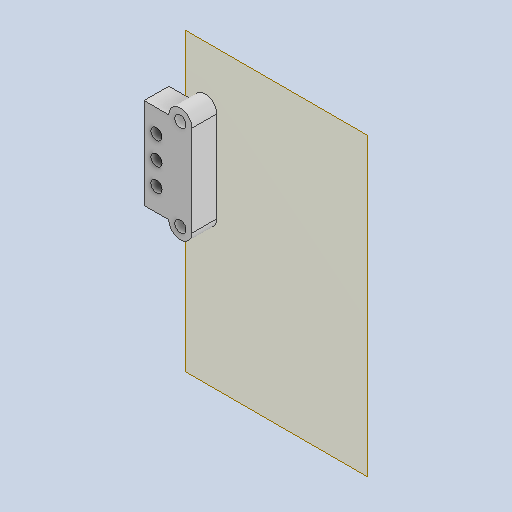
# Autodesk Inventor part: _idle_adt
Saved by Autodesk Inventor 2024.3 (Build 283343000, 343)
## iProperties
Created: 2024-09-05
Part Number: _idle_adt
Material: 일반
Document SubType Name: Modeling
Designer: gretc
Density: 1 g/cm^3
Appearance: 기본값
Author: gretc
Autodesk Inventor part; units mm, degrees
ref_plane "YZ Plane" through (0, 0, 0) normal (1, 0, 0) x (0, 1, 0)
ref_plane "XZ Plane" through (0, 0, 0) normal (0, 1, 0) x (-1, 0, 0)
ref_plane "XY Plane" through (0, 0, 0) normal (0, 0, 1) x (1, 0, 0)
ref_plane "작업 평면1" through (0, 0, 0) normal (0, 0, 1) x (1, 0, 0)
sketch "스케치1" plane through (0, 0, 0) normal (0, 0, 1) x (1, 0, 0)
  line L0 (-15, 14.5) -> (-11.5, 14.5) projected
  line L1 (-15, 14.5) -> (-20.1, 8.5) projected
  line L2 (-20.1, 8.5) -> (-20.1, -44.6) projected
  line L3 (-20.1, -44.6) -> (-15, -50.6) projected
  line L4 (-15, -50.6) -> (15, -50.6) projected
  line L5 (15, -50.6) -> (20.1, -44.6) projected
  line L6 (20.1, -44.6) -> (20.1, 8.5) projected
  line L7 (20.1, 8.5) -> (15, 14.5) projected
  line L8 (11.5, 14.5) -> (15, 14.5) projected
  arc A0 (14.5, 11.5) -> (11.5, 14.5) centre (11.5, 11.5) ccw projected
  line L9 (14.5, -42) -> (14.5, 11.5) projected
  arc A1 (11.5, -45) -> (14.5, -42) centre (11.5, -42) ccw projected
  line L10 (-11.5, -45) -> (11.5, -45) projected
  arc A2 (-14.5, -42) -> (-11.5, -45) centre (-11.5, -42) ccw projected
  line L11 (-14.5, 11.5) -> (-14.5, -42) projected
  arc A3 (-11.5, 14.5) -> (-14.5, 11.5) centre (-11.5, 11.5) ccw projected
  circle A4 centre (17.3, 4) radius 1.35 projected
  circle A5 centre (17.3, -18) radius 1.35 projected
  circle A6 centre (17.3, -40) radius 1.35 projected
  circle A7 centre (11, -47.8) radius 1.35 projected
  circle A8 centre (-17.3, 4) radius 1.35 projected
  circle A9 centre (-17.3, -18) radius 1.35 projected
  circle A10 centre (-17.3, -40) radius 1.35 projected
  circle A11 centre (-11, -47.8) radius 1.35 projected
  circle A12 centre (-17.3, -18) radius 2.8
  circle A13 centre (-17.3, 4) radius 2.8
  line L12 (-20.1, -18) -> (-20.1, 4)
  line L13 (-20.1, 4) -> (-26.1, 4)
  line L14 (-26.1, 4) -> (-26.1, -18)
  line L15 (-26.1, -18) -> (-20.1, -18)
  line L16 (-26.1, -18) -> (-26.1, -7)
  line L17 (-23.1, -18) -> (-23.1, -12.5)
  line L18 (-23.1, 4) -> (-23.1, -1.5)
  line L19 (-23.1, -1.5) -> (-23.1, -7)
  circle A14 centre (-23.1, -12.5) radius 1.35
  circle A15 centre (-23.1, -7) radius 1.35
  circle A16 centre (-23.1, -1.5) radius 1.35
  point P0 (0, 0)
  point P1 (-14.5, -18)
  point P2 (-14.5, 4)
  dimension "d0" = 6
  dimension "d1" = 11
  dimension "d2" = 5.5
  dimension "d3" = 2.7
  dimension "d4" = 2.7
  dimension "d5" = 2.7
  constraints: 16 end point, 6 coincident, 6 vertical, 3 centre point, 3 midpoint, 3 point on line, 2 parallel, 1 collinear, 1 perpendicular, 6 other
  measures "d0" distance of L13.end L12.end
  measures "d1" distance of L14.end L16.end
  measures "d2" distance of L18.start L18.end
  measures "d3" diameter of A14
  measures "d4" diameter of A15
  measures "d5" diameter of A16
extrude "돌출1" add sketch "스케치1" along normal blind 6 contours A13 L11 A12 L2 | A13 | L2 L15 L14 L13 | A12
